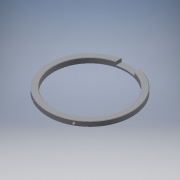
# Autodesk Inventor part: KE-SP-02-P1
Saved by Autodesk Inventor 2016 (Build 200138000, 138)
## iProperties
Created: 2015-08-04
Part Number: KE-SP-02-P1
Material: 一般
Document SubType Name: Modeling
Designer: ERIC
Density: 1 g/cm^3
Appearance: 預設
Author: ERIC
Autodesk Inventor part; units mm, degrees
sketch "草圖1" plane through (0, 0, 0) normal (0, 0, 1) x (1, 0, 0)
  circle A0 centre (0, 0) radius 49.85
  circle A1 centre (0, 0) radius 43
  dimension "d0" = 99.7
  dimension "d3" = 86
  constraints: 2 centre point, 2 coincident
  measures "d0" diameter of A0
  measures "d3" diameter of A1
extrude "擠出1" add sketch "草圖1" along normal blind 6
sketch "草圖2" plane through (0, 0, 6) normal (0, 0, 1) x (1, 0, 0)
  circle A0 centre (0, 0) radius 43 projected
  circle A1 centre (0, 0) radius 49.85 projected
  line L0 (0, 0) -> (0, 49.85)
  line L1 (11, 48.6212) -> (11, 41.5692)
  line L2 (-11, 48.6212) -> (-11, 41.5692)
  dimension "d6" = 22
  constraints: 6 end point, 5 point on circle, 2 parallel, 1 vertical, 1 other
  measures "d6" distance between parallel lines of L1 L2
extrude "擠出2" cut sketch "草圖2" against normal blind 4 contours A0 L0 A1 L1 | L2 A1 L0 A0
ref_plane "工作平面1" through (0, 0, 3) normal (0, 0, 1) x (1, 0, 0)
sketch "草圖3" plane through (0, 0, 3) normal (0, 0, 1) x (1, 0, 0)
  line L0 (0, 0) -> (0, -42.4806)
  line L1 (0, 0) -> (-25.5, -42.8342)
  line L2 (0, 0) -> (25.5, -42.8342)
  arc A0 (-11, 48.6212) -> (11, 48.6212) centre (0, 0) ccw projected
  line L3 (-25.5, -42.8342) -> (25.5, -42.8342)
  dimension "d9" = 51
  dimension "d27" = 61.532
  dimension "d28" = 30.766
  dimension "d29" = 30.766
  constraints: 8 end point, 2 point on circle, 1 perpendicular, 1 vertical, 1 other
  measures "d9" distance of L1.end L2.end
  measures "d27" angle of L1 L2
  measures "d28" angle of L0 L2
  measures "d29" angle of L1 L0
ref_plane "工作平面2" through (25.5, -42.8342, 3) normal (0.5115346, -0.8592627, 0) x (0.8592627, 0.5115346, 0)
ref_plane "工作平面3" through (-25.5, -42.8342, 3) normal (-0.5115346, -0.8592627, 0) x (0.8592627, -0.5115346, 0)
sketch "草圖4" plane through (25.5, -42.8342, 3) normal (0.5115346, -0.8592627, 0) x (0.8592627, 0.5115346, 0)
  point P0 (0, -3)
  point P1 (0, 0)
hole "孔1" at (25.5, -42.8342, 3) direction (-0.5115346, 0.8592627, 0) diameter 3 depth 2.5 tip angle 118
sketch "草圖5" plane through (-25.5, -42.8342, 3) normal (-0.5115346, -0.8592627, 0) x (0.8592627, -0.5115346, 0)
  point P0 (0, -3)
  point P1 (0, 0)
hole "孔2" at (-25.5, -42.8342, 3) direction (0.5115346, 0.8592627, 0) diameter 3 depth 2.5 tip angle 118
chamfer "倒角1" distance 0.5 angle 45 5 edges at (-26.2298, -34.0735, 6) (34.0735, 26.2298, 6) (-49.85, 0, 0) (-31.1181, -38.9447, 6) (38.9447, 31.1181, 6)
